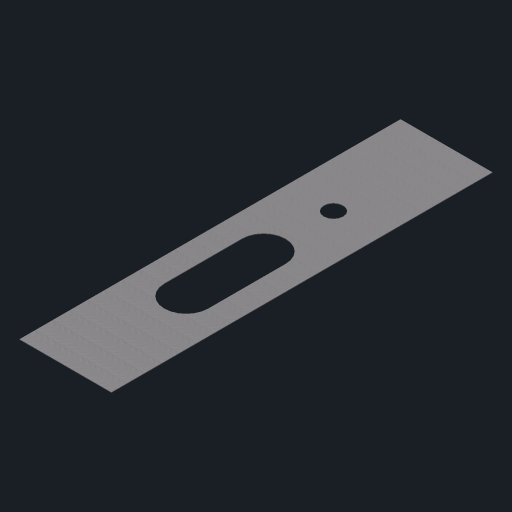
# Autodesk Inventor part: CHAPA_1
Saved by Autodesk Inventor 2024.3 (Build 283343000, 343)
## iProperties
Created: 2024-06-14
Part Number: CHAPA_1
Material: Steel, Mild, Welded
Document SubType Name: Sheet Metal
Designer: Niler
Density: 7.85 g/cm^3
Sheet Metal Rule: Default_mm
Appearance: Weld - Steel Mild
Flat Pattern Width: 23.7 cm
Flat Pattern Length: 98.3 cm
Flat Pattern Area: 2329.71 cm^2
Sheet Metal Width: 237.000 mm
Sheet Metal Length: 983.000 mm
Sheet Metal Area: 232971.000 mm^2
Author: Niler
Autodesk Inventor part; units mm, degrees
ref_plane "YZ Plane" through (0, 0, 0) normal (1, 0, 0) x (0, 1, 0)
ref_plane "XZ Plane" through (0, 0, 0) normal (0, 1, 0) x (-1, 0, 0)
ref_plane "XY Plane" through (0, 0, 0) normal (0, 0, 1) x (1, 0, 0)
sketch "Sketch1" plane through (0, 0, 0) normal (0, 1, 0) x (-1, 0, 0)
  line L0 (-118.5, 491.5) -> (118.5, 491.5)
  line L1 (118.5, 491.5) -> (118.5, -491.5)
  line L2 (118.5, -491.5) -> (-118.5, -491.5)
  line L3 (-118.5, -491.5) -> (-118.5, 491.5)
  line L4 (-118.5, 491.5) -> (118.5, -491.5) construction
  line L5 (118.5, 491.5) -> (-118.5, -491.5) construction
  point P0 (0, 0)
  dimension "d0" = 983
  dimension "d1" = 237
extrude "Plate1" add sketch "Sketch1" along normal blind 1.5
sketch "Sketch2" plane through (0, 1.5, 0) normal (0, 1, 0) x (1, 0, 0)
  line L0 (0, -180) -> (0, 20) construction
  line L1 (56.5, -180) -> (56.5, 20)
  line L2 (-56.5, 20) -> (-56.5, -180)
  arc A0 (-56.5, -180) -> (56.5, -180) centre (0, -180) ccw
  arc A1 (56.5, 20) -> (-56.5, 20) centre (0, 20) ccw
  line L3 (118.5, -491.5) -> (-118.5, -491.5) projected
  line L4 (118.5, 491.5) -> (118.5, -491.5) projected
  line L5 (-118.5, 491.5) -> (118.5, 491.5) projected
  line L6 (-118.5, -491.5) -> (-118.5, 491.5) projected
  line L7 (118.5, -491.5) -> (-118.5, -491.5) projected
  circle A2 centre (0, 200) radius 25
  point P0 (0, -80)
  point P1 (0, 76.5)
  point P2 (0, -236.5)
  point P3 (0, -491.5)
  point P4 (0, 0)
  point P5 (0, 0)
  point P6 (118.5, 0)
  point P7 (0, 491.5)
  dimension "d17" = 113
  dimension "d19" = 200
  dimension "d20" = 80
  dimension "d21" = 50
  dimension "d22" = 200
  constraints: 8 end point, 6 point on circle, 4 midpoint, 4 tangent, 3 centre point, 3 vertical alignment, 1 coincident, 1 horizontal alignment, 1 parallel, 1 vertical
  measures "d17" distance between parallel lines of L1 L2
  measures "d19" distance of L0.start L0.end
  measures "d20" distance of point (0, -80) point (0, 0)
  measures "d21" diameter of A2
  measures "d22" distance of A2.centre point (0, 0)
extrude "Extrusion1" cut sketch "Sketch2" against normal through all contours A0 L2 A1 L1 | A2
equation "\"d2\" = Thickness"
equation "\"BendRadius\" = Thickness"
equation "\"BendReliefWidth\" = Thickness"
equation "\"BendReliefDepth\" = 0.5 * Thickness"
equation "\"CornerReliefSize\" = 4 * Thickness"
equation "\"MinimumRemnant\" = 2 * Thickness"
equation "\"TransitionRadius\" = BendRadius"
equation "\"JacobiRadiusSize\" = BendRadius"
equation "\"GapSize\" = Thickness"
equation "\"Thickness\" = 1.5"
body "Solid1"
